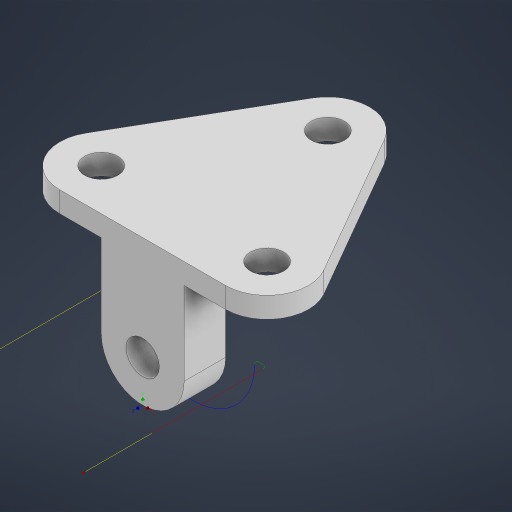
# Autodesk Inventor part: Table Holder
Saved by Autodesk Inventor 2023 (Build 270158000, 158)
## iProperties
Created: 2022-05-02
Part Number: Table Holder
Material: Generic
Document SubType Name: Modeling
Designer: FizzyApple12
Density: 1 g/cm^3
Appearance: Default
Author: FizzyApple12
Autodesk Inventor part; units mm, degrees
ref_plane "YZ Plane" through (0, 0, 0) normal (1, 0, 0) x (0, 1, 0)
ref_plane "XZ Plane" through (0, 0, 0) normal (0, 1, 0) x (-1, 0, 0)
ref_plane "XY Plane" through (0, 0, 0) normal (0, 0, 1) x (1, 0, 0)
sketch "Sketch1" plane through (0, 0, 0) normal (0, 0, 1) x (1, 0, 0)
  circle A0 centre (0, 0) radius 6.35
  line L0 (-6.35, 0) -> (-6.35, 12.7)
  line L1 (-6.35, 12.7) -> (6.35, 12.7)
  line L2 (6.35, 12.7) -> (6.35, 0)
  dimension "d0" = 12.7
  dimension "d1" = 12.7
  constraints: 6 end point, 2 coincident, 2 point on circle, 2 tangent, 1 centre point, 1 parallel, 1 perpendicular, 1 vertical
  measures "d0" diameter of A0
  measures "d1" distance of L0.start L0.end
extrude "Extrusion1" add sketch "Sketch1" along normal blind 6.35
hole "Hole1" at (0, 0, 0) direction (0, 0, 1) diameter 5.1054 end through all clearance for "Flat Head Machine Screw (82)" size "#10" standard "Ansi Unified Screw Threads"
sketch "Sketch2" plane through (-6.35, 12.7, 0) normal (0, 1, 0) x (1, 0, 0)
  line L0 (6.35, 0) -> (19.05, 0) construction
  line L1 (6.35, 0) -> (-6.35, 0) construction
  line L2 (-6.35, 0) -> (6.35, 21.997) construction
  line L3 (6.35, 21.997) -> (19.05, 0) construction
  circle A0 centre (19.05, 0) radius 6.35 construction
  circle A1 centre (-6.35, 0) radius 6.35 construction
  circle A2 centre (6.35, 21.997) radius 6.35 construction
  line L4 (0.8507, 25.172) -> (-11.8493, 3.175)
  line L5 (11.8493, 25.172) -> (24.5493, 3.175)
  line L6 (19.05, -6.35) -> (12.7, -6.35)
  line L7 (0, -6.35) -> (12.7, -6.35) projected
  line L8 (12.7, -6.35) -> (0, -6.35)
  line L9 (0, -6.35) -> (-6.35, -6.35)
  arc A3 (-11.8493, 3.175) -> (-6.35, -6.35) centre (-6.35, 0) ccw
  arc A4 (11.8493, 25.172) -> (0.8507, 25.172) centre (6.35, 21.997) ccw
  arc A5 (19.05, -6.35) -> (24.5493, 3.175) centre (19.05, 0) ccw
  dimension "d11" = 12.7
  dimension "d12" = 12.7
  dimension "d13" = 25.4
  dimension "d14" = 25.4
  dimension "d15" = 12.7
  dimension "d16" = 12.7
  dimension "d17" = 12.7
  constraints: 18 end point, 12 point on circle, 10 tangent, 6 centre point, 6 coincident, 2 horizontal, 1 collinear, 1 point on line
  measures "d11" distance of L0.start L0.end
  measures "d12" distance of L0.start L1.end
  measures "d13" distance of L1.end L2.end
  measures "d14" distance of L0.end L2.end
  measures "d15" diameter of A0
  measures "d16" diameter of A1
  measures "d17" diameter of A2
extrude "Extrusion2" add sketch "Sketch2" along normal blind 3.175
hole "Hole2" at (12.7, 12.7, 0) at (0, 12.7, -21.997) at (-12.7, 12.7, 0) direction (0, 1, 0) diameter 5.1054 end through all clearance for "Flat Head Machine Screw (82)" size "#10" standard "Ansi Unified Screw Threads"
body "Solid1"
